Autodesk Inventor part; units mm, degrees
(part 3 of 3)
  line L610 (-443.23, 622.6009) -> (-468.63, 637.2656)
  arc A722 (-468.63, 646.0644) -> (-468.63, 637.2656) centre (-466.09, 641.665) ccw
  line L611 (-479.425, 655.9631) -> (-479.425, 685.2925)
  arc A723 (-471.805, 689.6919) -> (-479.425, 685.2925) centre (-474.345, 685.2925) ccw
  line L612 (-471.805, 689.6919) -> (-446.405, 675.0272)
  arc A724 (-446.405, 666.2284) -> (-446.405, 675.0272) centre (-448.945, 670.6278) ccw
  line L613 (-446.405, 666.2284) -> (-471.805, 651.5637)
  arc A725 (-479.425, 655.9631) -> (-471.805, 651.5637) centre (-474.345, 655.9631) ccw
  line L614 (-493.395, 651.5637) -> (-518.795, 666.2284)
  arc A726 (-518.795, 675.0272) -> (-518.795, 666.2284) centre (-516.255, 670.6278) ccw
  line L615 (-518.795, 675.0272) -> (-493.395, 689.6919)
  arc A727 (-485.775, 685.2925) -> (-493.395, 689.6919) centre (-490.855, 685.2925) ccw
  line L616 (-485.775, 685.2925) -> (-485.775, 655.9631)
  arc A728 (-493.395, 651.5637) -> (-485.775, 655.9631) centre (-490.855, 655.9631) ccw
  line L617 (-468.63, 530.2133) -> (-443.23, 544.878)
  line L618 (-443.23, 506.7498) -> (-468.63, 521.4145)
  arc A729 (-468.63, 530.2133) -> (-468.63, 521.4145) centre (-466.09, 525.8139) ccw
  arc A730 (-435.61, 540.4786) -> (-443.23, 544.878) centre (-440.69, 540.4786) ccw
  line L619 (-435.61, 540.4786) -> (-435.61, 511.1492)
  arc A731 (-443.23, 506.7498) -> (-435.61, 511.1492) centre (-440.69, 511.1492) ccw
  line L620 (-479.425, 540.112) -> (-479.425, 569.4414)
  line L621 (-446.405, 550.3772) -> (-471.805, 535.7126)
  arc A732 (-479.425, 540.112) -> (-471.805, 535.7126) centre (-474.345, 540.112) ccw
  arc A733 (-471.805, 573.8408) -> (-479.425, 569.4414) centre (-474.345, 569.4414) ccw
  line L622 (-471.805, 573.8408) -> (-446.405, 559.1761)
  arc A734 (-446.405, 550.3772) -> (-446.405, 559.1761) centre (-448.945, 554.7767) ccw
  line L623 (-493.395, 535.7126) -> (-518.795, 550.3772)
  line L624 (-485.775, 569.4414) -> (-485.775, 540.112)
  arc A735 (-493.395, 535.7126) -> (-485.775, 540.112) centre (-490.855, 540.112) ccw
  arc A736 (-518.795, 559.1761) -> (-518.795, 550.3772) centre (-516.255, 554.7767) ccw
  line L625 (-518.795, 559.1761) -> (-493.395, 573.8408)
  arc A737 (-485.775, 569.4414) -> (-493.395, 573.8408) centre (-490.855, 569.4414) ccw
  line L626 (-496.57, 521.4145) -> (-521.97, 506.7498)
  line L627 (-521.97, 544.878) -> (-496.57, 530.2133)
  arc A738 (-496.57, 521.4145) -> (-496.57, 530.2133) centre (-499.11, 525.8139) ccw
  arc A739 (-529.59, 511.1492) -> (-521.97, 506.7498) centre (-524.51, 511.1492) ccw
  line L628 (-529.59, 511.1492) -> (-529.59, 540.4786)
  arc A740 (-521.97, 544.878) -> (-529.59, 540.4786) centre (-524.51, 540.4786) ccw
  line L629 (-485.775, 511.5158) -> (-485.775, 482.1864)
  line L630 (-518.795, 501.2505) -> (-493.395, 515.9152)
  arc A741 (-485.775, 511.5158) -> (-493.395, 515.9152) centre (-490.855, 511.5158) ccw
  arc A742 (-493.395, 477.787) -> (-485.775, 482.1864) centre (-490.855, 482.1864) ccw
  line L631 (-493.395, 477.787) -> (-518.795, 492.4517)
  arc A743 (-518.795, 501.2505) -> (-518.795, 492.4517) centre (-516.255, 496.8511) ccw
  line L632 (-418.465, 501.2505) -> (-393.065, 515.9152)
  arc A744 (-418.465, 501.2505) -> (-418.465, 492.4517) centre (-415.925, 496.8511) ccw
  line L633 (-393.065, 477.787) -> (-418.465, 492.4517)
  arc A745 (-393.065, 477.787) -> (-385.445, 482.1864) centre (-390.525, 482.1864) ccw
  line L634 (-385.445, 511.5158) -> (-385.445, 482.1864)
  arc A746 (-385.445, 511.5158) -> (-393.065, 515.9152) centre (-390.525, 511.5158) ccw
  line L635 (-429.26, 511.1492) -> (-429.26, 540.4786)
  arc A747 (-429.26, 511.1492) -> (-421.64, 506.7498) centre (-424.18, 511.1492) ccw
  line L636 (-396.24, 521.4145) -> (-421.64, 506.7498)
  arc A748 (-396.24, 521.4145) -> (-396.24, 530.2133) centre (-398.78, 525.8139) ccw
  line L637 (-421.64, 544.878) -> (-396.24, 530.2133)
  arc A749 (-421.64, 544.878) -> (-429.26, 540.4786) centre (-424.18, 540.4786) ccw
  line L638 (-443.23, 506.7498) -> (-468.63, 521.4145)
  arc A750 (-443.23, 506.7498) -> (-435.61, 511.1492) centre (-440.69, 511.1492) ccw
  line L639 (-435.61, 540.4786) -> (-435.61, 511.1492)
  arc A751 (-435.61, 540.4786) -> (-443.23, 544.878) centre (-440.69, 540.4786) ccw
  line L640 (-468.63, 530.2133) -> (-443.23, 544.878)
  arc A752 (-468.63, 530.2133) -> (-468.63, 521.4145) centre (-466.09, 525.8139) ccw
  line L641 (-446.405, 492.4517) -> (-471.805, 477.787)
  arc A753 (-446.405, 492.4517) -> (-446.405, 501.2505) centre (-448.945, 496.8511) ccw
  line L642 (-471.805, 515.9152) -> (-446.405, 501.2505)
  arc A754 (-471.805, 515.9152) -> (-479.425, 511.5158) centre (-474.345, 511.5158) ccw
  line L643 (-479.425, 482.1864) -> (-479.425, 511.5158)
  arc A755 (-479.425, 482.1864) -> (-471.805, 477.787) centre (-474.345, 482.1864) ccw
  line L644 (-435.61, 482.553) -> (-435.61, 453.2236)
  arc A756 (-435.61, 482.553) -> (-443.23, 486.9524) centre (-440.69, 482.553) ccw
  line L645 (-468.63, 472.2877) -> (-443.23, 486.9524)
  arc A757 (-468.63, 472.2877) -> (-468.63, 463.4889) centre (-466.09, 467.8883) ccw
  line L646 (-443.23, 448.8242) -> (-468.63, 463.4889)
  arc A758 (-443.23, 448.8242) -> (-435.61, 453.2236) centre (-440.69, 453.2236) ccw
  circle A759 centre (-432.435, 554.7767) radius 11.43
  arc A760 (-435.61, 540.4786) -> (-443.23, 544.878) centre (-440.69, 540.4786) ccw
  line L647 (-435.61, 540.4786) -> (-435.61, 511.1492)
  arc A761 (-443.23, 506.7498) -> (-435.61, 511.1492) centre (-440.69, 511.1492) ccw
  line L648 (-443.23, 506.7498) -> (-468.63, 521.4145)
  arc A762 (-468.63, 530.2133) -> (-468.63, 521.4145) centre (-466.09, 525.8139) ccw
  line L649 (-468.63, 530.2133) -> (-443.23, 544.878)
  arc A763 (-421.64, 544.878) -> (-429.26, 540.4786) centre (-424.18, 540.4786) ccw
  line L650 (-421.64, 544.878) -> (-396.24, 530.2133)
  arc A764 (-396.24, 521.4145) -> (-396.24, 530.2133) centre (-398.78, 525.8139) ccw
  line L651 (-396.24, 521.4145) -> (-421.64, 506.7498)
  arc A765 (-429.26, 511.1492) -> (-421.64, 506.7498) centre (-424.18, 511.1492) ccw
  line L652 (-429.26, 511.1492) -> (-429.26, 540.4786)
  arc A766 (-418.465, 559.1761) -> (-418.465, 550.3772) centre (-415.925, 554.7767) ccw
  line L653 (-418.465, 559.1761) -> (-393.065, 573.8408)
  arc A767 (-385.445, 569.4414) -> (-393.065, 573.8408) centre (-390.525, 569.4414) ccw
  line L654 (-385.445, 569.4414) -> (-385.445, 540.112)
  arc A768 (-393.065, 535.7126) -> (-385.445, 540.112) centre (-390.525, 540.112) ccw
  line L655 (-393.065, 535.7126) -> (-418.465, 550.3772)
  arc A769 (-429.26, 569.0747) -> (-421.64, 564.6753) centre (-424.18, 569.0747) ccw
  line L656 (-429.26, 569.0747) -> (-429.26, 598.4041)
  arc A770 (-421.64, 602.8035) -> (-429.26, 598.4041) centre (-424.18, 598.4041) ccw
  line L657 (-421.64, 602.8035) -> (-396.24, 588.1388)
  arc A771 (-396.24, 579.34) -> (-396.24, 588.1388) centre (-398.78, 583.7394) ccw
  line L658 (-396.24, 579.34) -> (-421.64, 564.6753)
  arc A772 (-443.23, 564.6753) -> (-435.61, 569.0747) centre (-440.69, 569.0747) ccw
  line L659 (-443.23, 564.6753) -> (-468.63, 579.34)
  arc A773 (-468.63, 588.1388) -> (-468.63, 579.34) centre (-466.09, 583.7394) ccw
  line L660 (-468.63, 588.1388) -> (-443.23, 602.8035)
  arc A774 (-435.61, 598.4041) -> (-443.23, 602.8035) centre (-440.69, 598.4041) ccw
  line L661 (-435.61, 598.4041) -> (-435.61, 569.0747)
  circle A775 centre (-432.435, 612.7022) radius 11.43
  line L662 (-385.445, 627.3669) -> (-385.445, 598.0375)
  arc A776 (-393.065, 593.6381) -> (-385.445, 598.0375) centre (-390.525, 598.0375) ccw
  line L663 (-393.065, 593.6381) -> (-418.465, 608.3028)
  arc A777 (-418.465, 617.1016) -> (-418.465, 608.3028) centre (-415.925, 612.7022) ccw
  line L664 (-418.465, 617.1016) -> (-393.065, 631.7663)
  arc A778 (-385.445, 627.3669) -> (-393.065, 631.7663) centre (-390.525, 627.3669) ccw
  line L665 (-421.64, 660.7291) -> (-396.24, 646.0644)
  arc A779 (-396.24, 637.2656) -> (-396.24, 646.0644) centre (-398.78, 641.665) ccw
  line L666 (-396.24, 637.2656) -> (-421.64, 622.6009)
  arc A780 (-429.26, 627.0003) -> (-421.64, 622.6009) centre (-424.18, 627.0003) ccw
  line L667 (-429.26, 627.0003) -> (-429.26, 656.3297)
  arc A781 (-421.64, 660.7291) -> (-429.26, 656.3297) centre (-424.18, 656.3297) ccw
  line L668 (-468.63, 646.0644) -> (-443.23, 660.7291)
  arc A782 (-435.61, 656.3297) -> (-443.23, 660.7291) centre (-440.69, 656.3297) ccw
  line L669 (-435.61, 656.3297) -> (-435.61, 627.0003)
  arc A783 (-443.23, 622.6009) -> (-435.61, 627.0003) centre (-440.69, 627.0003) ccw
  line L670 (-443.23, 622.6009) -> (-468.63, 637.2656)
  arc A784 (-468.63, 646.0644) -> (-468.63, 637.2656) centre (-466.09, 641.665) ccw
  line L671 (-479.425, 598.0375) -> (-479.425, 627.3669)
  arc A785 (-471.805, 631.7663) -> (-479.425, 627.3669) centre (-474.345, 627.3669) ccw
  line L672 (-471.805, 631.7663) -> (-446.405, 617.1016)
  arc A786 (-446.405, 608.3028) -> (-446.405, 617.1016) centre (-448.945, 612.7022) ccw
  line L673 (-446.405, 608.3028) -> (-471.805, 593.6381)
  arc A787 (-479.425, 598.0375) -> (-471.805, 593.6381) centre (-474.345, 598.0375) ccw
  line L674 (-443.23, 564.6753) -> (-468.63, 579.34)
  arc A788 (-468.63, 588.1388) -> (-468.63, 579.34) centre (-466.09, 583.7394) ccw
  line L675 (-468.63, 588.1388) -> (-443.23, 602.8035)
  arc A789 (-435.61, 598.4041) -> (-443.23, 602.8035) centre (-440.69, 598.4041) ccw
  line L676 (-435.61, 598.4041) -> (-435.61, 569.0747)
  arc A790 (-443.23, 564.6753) -> (-435.61, 569.0747) centre (-440.69, 569.0747) ccw
  circle A791 centre (-433.5961, 671.2379) radius 11.43
  point P0 (0, 0)
  point P1 (-398.9917, 381)
  point P2 (-385.445, 357.5365)
  point P3 (-426.085, 381)
  point P4 (-385.445, 404.4635)
  point P5 (-388.62, 409.9628)
  point P6 (-429.26, 386.4993)
  point P7 (-429.26, 433.4263)
  point P8 (-435.61, 433.4263)
  point P9 (-435.61, 386.4993)
  point P10 (-476.25, 409.9628)
  point P11 (-479.425, 404.4635)
  point P12 (-438.785, 381)
  point P13 (-479.425, 357.5365)
  point P14 (-476.25, 352.0372)
  point P15 (-435.61, 375.5007)
  point P16 (-435.61, 328.5737)
  point P17 (-429.26, 328.5737)
  point P18 (-429.26, 375.5007)
  point P19 (-388.62, 352.0372)
  point P20 (-450.3275, 367.0036)
  point P21 (-479.425, 299.6109)
  point P22 (-438.785, 323.0744)
  point P23 (-479.425, 346.538)
  point P24 (-479.425, 329.5436)
  point P25 (-435.61, 270.6482)
  point P26 (-435.61, 317.5752)
  point P27 (-476.25, 294.1117)
  point P28 (-461.5325, 285.6145)
  point P29 (-388.62, 294.1117)
  point P30 (-429.26, 317.5752)
  point P31 (-429.26, 270.6482)
  point P32 (-414.5425, 279.1453)
  point P33 (-385.445, 346.538)
  point P34 (-426.085, 323.0744)
  point P35 (-385.445, 299.6109)
  point P36 (-385.445, 316.6053)
  point P37 (-429.26, 375.5007)
  point P38 (-429.26, 328.5737)
  point P39 (-388.62, 352.0372)
  point P40 (-403.3375, 360.5344)
  point P41 (-438.785, 265.1489)
  point P42 (-479.425, 288.6124)
  point P43 (-479.425, 241.6854)
  point P44 (-464.7075, 250.1825)
  point P45 (-435.61, 259.6496)
  point P46 (-476.25, 236.1861)
  point P47 (-435.61, 212.7226)
  point P48 (-435.61, 229.7169)
  point P49 (-429.26, 259.6496)
  point P50 (-429.26, 212.7226)
  point P51 (-388.62, 236.1861)
  point P52 (-403.3375, 244.6833)
  point P53 (-426.085, 265.1489)
  point P54 (-385.445, 241.6854)
  point P55 (-385.445, 288.6124)
  point P56 (-400.1625, 280.1153)
  point P57 (-429.26, 270.6482)
  point P58 (-388.62, 294.1117)
  point P59 (-429.26, 317.5752)
  point P60 (-429.26, 300.5809)
  point P61 (-453.5025, 215.7205)
  point P62 (-479.425, 230.6869)
  point P63 (-438.785, 207.2233)
  point P64 (-479.425, 183.7598)
  point P65 (-450.3275, 193.2269)
  point P66 (-476.25, 178.2606)
  point P67 (-435.61, 201.7241)
  point P68 (-435.61, 154.7971)
  point P69 (-429.26, 184.7298)
  point P70 (-429.26, 154.7971)
  point P71 (-429.26, 201.7241)
  point P72 (-388.62, 178.2606)
  point P73 (-411.3675, 198.7262)
  point P74 (-385.445, 183.7598)
  point P75 (-426.085, 207.2233)
  point P76 (-385.445, 230.6869)
  point P77 (-414.5425, 221.2198)
  point P78 (-388.62, 236.1861)
  point P79 (-429.26, 212.7226)
  point P80 (-429.26, 259.6496)
  point P81 (-479.425, 125.8343)
  point P82 (-438.785, 149.2978)
  point P83 (-479.425, 172.7613)
  point P84 (-479.425, 155.767)
  point P85 (-435.61, 96.8715)
  point P86 (-435.61, 143.7985)
  point P87 (-476.25, 120.335)
  point P88 (-461.5325, 111.8379)
  point P89 (-388.62, 120.335)
  point P90 (-429.26, 143.7985)
  point P91 (-429.26, 96.8715)
  point P92 (-414.5425, 105.3687)
  point P93 (-385.445, 172.7613)
  point P94 (-426.085, 149.2978)
  point P95 (-385.445, 125.8343)
  point P96 (-385.445, 142.8286)
  point P97 (-429.26, 201.7241)
  point P98 (-429.26, 154.7971)
  point P99 (-388.62, 178.2606)
  point P100 (-403.3375, 186.7577)
  point P101 (-435.61, 143.7985)
  point P102 (-435.61, 96.8715)
  point P103 (-435.61, 113.8658)
  point P104 (-476.25, 120.335)
  point P105 (-479.425, 114.8358)
  point P106 (-438.785, 91.3722)
  point P107 (-453.5025, 99.8694)
  point P108 (-479.425, 67.9087)
  point P109 (-476.25, 62.4095)
  point P110 (-435.61, 85.873)
  point P111 (-450.3275, 77.3758)
  point P112 (-435.61, 38.9459)
  point P113 (-429.26, 38.9459)
  point P114 (-429.26, 85.873)
  point P115 (-429.26, 68.8787)
  point P116 (-388.62, 62.4095)
  point P117 (-385.445, 67.9087)
  point P118 (-426.085, 91.3722)
  point P119 (-411.3675, 82.8751)
  point P120 (-385.445, 114.8358)
  point P121 (-385.445, 56.9102)
  point P122 (-426.085, 33.4467)
  point P123 (-385.445, 9.9832)
  point P124 (-385.445, 26.9775)
  point P125 (-479.425, 9.9832)
  point P126 (-438.785, 33.4467)
  point P127 (-479.425, 56.9102)
  point P128 (-479.425, 39.9159)
  point P129 (-526.415, 91.3722)
  point P130 (-485.775, 67.9087)
  point P131 (-485.775, 114.8358)
  point P132 (-500.4925, 106.3386)
  point P133 (-529.59, 38.9459)
  point P134 (-488.95, 62.4095)
  point P135 (-529.59, 85.873)
  point P136 (-529.59, 68.8787)
  point P137 (-485.775, 9.9832)
  point P138 (-485.775, 56.9102)
  point P139 (-526.415, 33.4467)
  point P140 (-511.6975, 24.9495)
  point P141 (-438.785, 33.4467)
  point P142 (-479.425, 56.9102)
  point P143 (-479.425, 9.9832)
  point P144 (-464.7075, 18.4803)
  point P145 (-435.61, 85.873)
  point P146 (-476.25, 62.4095)
  point P147 (-435.61, 38.9459)
  point P148 (-435.61, 55.9403)
  point P149 (-485.775, 125.8343)
  point P150 (-526.415, 149.2978)
  point P151 (-511.6975, 140.8006)
  point P152 (-485.775, 172.7613)
  point P153 (-488.95, 120.335)
  point P154 (-529.59, 96.8715)
  point P155 (-514.8725, 105.3687)
  point P156 (-529.59, 143.7985)
  point P157 (-485.775, 114.8358)
  point P158 (-485.775, 67.9087)
  point P159 (-485.775, 84.903)
  point P160 (-526.415, 91.3722)
  point P161 (-479.425, 114.8358)
  point P162 (-438.785, 91.3722)
  point P163 (-453.5025, 99.8694)
  point P164 (-479.425, 67.9087)
  point P165 (-476.25, 120.335)
  point P166 (-435.61, 143.7985)
  point P167 (-450.3275, 135.3014)
  point P168 (-435.61, 96.8715)
  point P169 (-485.775, 67.9087)
  point P170 (-526.415, 91.3722)
  point P171 (-511.6975, 82.8751)
  point P172 (-485.775, 114.8358)
  point P173 (-488.95, 120.335)
  point P174 (-529.59, 96.8715)
  point P175 (-514.8725, 105.3687)
  point P176 (-529.59, 143.7985)
  point P177 (-535.94, 143.7985)
  point P178 (-535.94, 96.8715)
  point P179 (-535.94, 113.8658)
  point P180 (-576.58, 120.335)
  point P181 (-539.115, 149.2978)
  point P182 (-579.755, 125.8343)
  point P183 (-579.755, 172.7613)
  point P184 (-553.8325, 157.7949)
  point P185 (-586.105, 172.7613)
  point P186 (-586.105, 125.8343)
  point P187 (-626.745, 149.2978)
  point P188 (-600.8225, 164.2641)
  point P189 (-576.58, 120.335)
  point P190 (-535.94, 143.7985)
  point P191 (-550.6575, 135.3014)
  point P192 (-535.94, 96.8715)
  point P193 (-529.59, 96.8715)
  point P194 (-529.59, 143.7985)
  point P195 (-529.59, 126.8042)
  point P196 (-488.95, 120.335)
  point P197 (-485.775, 125.8343)
  point P198 (-526.415, 149.2978)
  point P199 (-511.6975, 140.8006)
  dimension "d168" = 5.08
  dimension "d169" = 25.4
  dimension "d172" = 360
  dimension "d177" = 10.16
  dimension "d179" = 381
  dimension "d183" = 360
  dimension "d185" = 10.16
  dimension "d186" = 25.4
  dimension "d189" = 360
  dimension "d193" = 360
  dimension "d197" = 360
  dimension "d201" = 360
  dimension "d205" = 120
  dimension "d209" = 60
  dimension "d211" = 6.35
  dimension "d212" = 9.6375
  dimension "d213" = 4.445
  dimension "d214" = 12.6077
  dimension "d216" = 368.9958
  dimension "d219" = 360
  dimension "d223" = 360
  dimension "d227" = 180
  dimension "d231" = 120
  dimension "d235" = 360
  dimension "d239" = 360
  dimension "d243" = 120
  dimension "d247" = 120
  dimension "d251" = 120
  dimension "d255" = 360
  dimension "d259" = 360
  dimension "d263" = 360
  dimension "d267" = 360
  dimension "d271" = 360
  dimension "d275" = 360
  dimension "d279" = 360
  dimension "d283" = 360
  dimension "d287" = 360
  dimension "d291" = 360
  dimension "d295" = 360
  dimension "d299" = 360
  dimension "d303" = 360
  dimension "d307" = 360
  dimension "d311" = 360
  dimension "d315" = 360
  dimension "d319" = 360
  dimension "d323" = 360
  dimension "d327" = 360
  dimension "d331" = 180
  dimension "d335" = 120
  dimension "d339" = 360
  dimension "d343" = 360
  dimension "d347" = 360
  dimension "d351" = 360
  dimension "d355" = 360
  dimension "d359" = 360
  dimension "d363" = 360
  dimension "d367" = 360
  dimension "d371" = 360
  dimension "d375" = 360
  dimension "d379" = 360
  constraints: 1511 point on line, 1330 end point, 1302 point on circle, 724 centre point, 102 tangent, 51 equal radius, 8 coincident, 4 horizontal alignment, 3 midpoint, 1 perpendicular, 1 vertical, 4970 other
  measures "d168" radius of A1
  measures "d169" horizontal distance of A1.centre A2.centre
  measures "d177" diameter of A24
  measures "d179" distance of L23.start L23.end
  measures "d185" diameter of A42
  measures "d186" distance between parallel lines of L46 L48
  measures "d211" distance between parallel lines of L15 L17
  measures "d212" horizontal distance of A17.centre point (-450.328, 367.004)
  measures "d213" distance between parallel lines of L3 L7
  measures "d214" diameter of A25
  measures "d216" distance of L24.start L24.end
body "Solid1"
